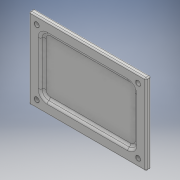
# Autodesk Inventor part: Solar Module Lid
Saved by Autodesk Inventor 2017 (Build 210142000, 142)
## iProperties
Created: 2019-06-21
Part Number: Solar Module Lid
Material: Generic
Document SubType Name: Modeling
Designer: harneet
Density: 1 g/cm^3
Appearance: Default
Author: harneet
Autodesk Inventor part; units mm, degrees
ref_plane "YZ Plane" through (0, 0, 0) normal (1, 0, 0) x (0, 1, 0)
ref_plane "XZ Plane" through (0, 0, 0) normal (0, 1, 0) x (-1, 0, 0)
ref_plane "XY Plane" through (0, 0, 0) normal (0, 0, 1) x (1, 0, 0)
sketch "Sketch1" plane through (0, 0, 0) normal (0, 1, 0) x (-1, 0, 0)
  line L0 (45, -31) -> (-45, -31)
  line L1 (-45, -31) -> (-45, 31)
  line L2 (-45, 31) -> (45, 31)
  line L3 (45, 31) -> (45, -31)
  circle A0 centre (39, -25) radius 1.75
  circle A1 centre (-39, -25) radius 1.75
  circle A2 centre (-39, 25) radius 1.75
  circle A3 centre (39, 25) radius 1.75
  point P0 (0, 0)
  dimension "d0" = 3.5
  dimension "d1" = 3.5
  dimension "d2" = 3.5
  dimension "d3" = 3.5
  dimension "d4" = 6
  dimension "d5" = 6
  dimension "d6" = 6
  dimension "d7" = 6
  dimension "d8" = 6
  dimension "d9" = 6
  dimension "d10" = 6
  dimension "d11" = 6
  dimension "d12" = 90
  dimension "d13" = 45
  dimension "d14" = 62
  dimension "d15" = 31
  constraints: 8 end point, 4 centre point, 2 parallel, 1 horizontal, 1 perpendicular
  measures "d0" diameter of A0
  measures "d1" diameter of A1
  measures "d2" diameter of A2
  measures "d3" diameter of A3
  measures "d4" distance from line of L2 A3.centre
  measures "d5" distance from line of A3.centre L3
  measures "d6" distance from line of A0.centre L0
  measures "d7" distance from line of A0.centre L3
  measures "d8" distance from line of L1 A1.centre
  measures "d9" distance from line of A1.centre L0
  measures "d10" distance from line of A2.centre L2
  measures "d11" distance from line of A2.centre L1
  measures "d12" distance of L1.end L2.end
  measures "d13" distance from line of L1 point (0, 0)
  measures "d14" distance between parallel lines of L2 L0
  measures "d15" distance from line of L0 point (0, 0)
extrude "Extrusion1" add sketch "Sketch1" along normal blind 4
sketch "Sketch2" plane through (0, 0, 0) normal (0, -1, 0) x (1, 0, 0)
  circle A0 centre (-39, 25) radius 1.75 projected
  circle A1 centre (39, 25) radius 1.75 projected
  circle A2 centre (39, -25) radius 1.75 projected
  circle A3 centre (-39, -25) radius 1.75 projected
  line L0 (-45, -31) -> (45, -31) projected
  line L1 (45, -31) -> (45, 31) projected
  line L2 (45, 31) -> (-45, 31) projected
  line L3 (-45, 31) -> (-45, -31) projected
  line L4 (-31, 22) -> (31, 22)
  line L5 (36, 17) -> (36, -17)
  line L6 (31, -22) -> (-31, -22)
  line L7 (-36, -17) -> (-36, 17)
  arc A4 (-31, 22) -> (-36, 17) centre (-31, 17) ccw
  arc A5 (-36, -17) -> (-31, -22) centre (-31, -17) ccw
  arc A6 (31, -22) -> (36, -17) centre (31, -17) ccw
  arc A7 (36, 17) -> (31, 22) centre (31, 17) ccw
  point P0 (0, 0)
  dimension "d18" = 5
  dimension "d19" = 5
  dimension "d20" = 9
  constraints: 8 end point, 8 point on circle, 8 tangent, 4 centre point, 2 equal radius, 3 other
  measures "d18" radius of A4
  measures "d19" radius of A5
  measures "d20" distance between parallel lines of L4 L2
extrude "Extrusion2" cut sketch "Sketch2" against normal blind 2.5 contours L4 A7 L5 A6 L6 A5 L7 A4
fillet "Fillet1" radius 2 16 edges at (0, 0, 22) (0, 2.5, 22) (34.5355, 0, 20.5355) (36, 0, 0) (34.5355, 0, -20.5355) (0, 0, -22) (-34.5355, 0, -20.5355) (-36, 0, 0) (-34.5355, 0, 20.5355) (34.5355, 2.5, 20.5355) (36, 2.5, 0) (34.5355, 2.5, -20.5355) (0, 2.5, -22) (-34.5355, 2.5, -20.5355) (-36, 2.5, 0) (-34.5355, 2.5, 20.5355)
fillet "Fillet2" radius 1 4 edges at (0, 4, -31) (-45, 4, 0) (0, 4, 31) (45, 4, 0)
fillet "Fillet3" radius 1 12 edges at (45, 1.5, 31) (45, 0, 0) (45, 1.5, -31) (44.7071, 3.7071, 30.7071) (44.7071, 3.7071, -30.7071) (0, 0, -31) (0, 0, 31) (-45, 0, 0) (-44.7071, 3.7071, -30.7071) (-45, 1.5, -31) (-44.7071, 3.7071, 30.7071) (-45, 1.5, 31)
fillet "Fillet4" radius 1 4 edges at (40.75, 4, 25) (-37.25, 4, 25) (-37.25, 4, -25) (40.75, 4, -25)
chamfer "Chamfer1" distance 0.2 angle 45 4 edges at (-37.25, 0, 25) (40.75, 0, 25) (40.75, 0, -25) (-37.25, 0, -25)
equation "\"d13\" = 0.5 * d12"
equation "\"d15\" = 0.5 * d14"
body "Solid1"
